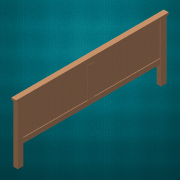
# Autodesk Inventor part: Footer
Saved by Autodesk Inventor 2017 (Build 210142000, 142)
## iProperties
Created: 2017-06-03
Part Number: Footer
Material: Wood (Cherry)
Document SubType Name: Modeling
Designer: Michael
Density: 0.63 g/cm^3
Appearance: Cherry - Natural Low Gloss
Author: Michael
Autodesk Inventor part; units mm, degrees
ref_plane "YZ Plane" through (0, 0, 0) normal (1, 0, 0) x (0, 1, 0)
ref_plane "XZ Plane" through (0, 0, 0) normal (0, 1, 0) x (-1, 0, 0)
ref_plane "XY Plane" through (0, 0, 0) normal (0, 0, 1) x (1, 0, 0)
sketch "Sketch1" plane through (0, 0, 0) normal (0, 1, 0) x (-1, 0, 0)
  line L0 (-23.8125, 804.8625) -> (23.8125, 804.8625)
  line L1 (23.8125, 804.8625) -> (23.8125, 746.125)
  line L2 (23.8125, 746.125) -> (-23.8125, 746.125)
  line L3 (-23.8125, 746.125) -> (-23.8125, 804.8625)
  line L4 (-23.8125, 804.8625) -> (23.8125, 746.125) construction
  line L5 (23.8125, 804.8625) -> (-23.8125, 746.125) construction
  line L6 (-23.8125, -746.125) -> (23.8125, -746.125)
  line L7 (23.8125, -746.125) -> (23.8125, -804.8625)
  line L8 (23.8125, -804.8625) -> (-23.8125, -804.8625)
  line L9 (-23.8125, -804.8625) -> (-23.8125, -746.125)
  line L10 (-23.8125, -746.125) -> (23.8125, -804.8625) construction
  line L11 (23.8125, -746.125) -> (-23.8125, -804.8625) construction
  line L12 (0, 746.125) -> (0, 0) construction
  line L13 (0, 0) -> (0, -746.125) construction
  point P0 (0, 775.4938)
  point P1 (0, -775.4938)
  point P2 (0, 775.4938)
  point P3 (0, -775.4938)
  dimension "d0" = 47.625
  dimension "d1" = 58.7375
  dimension "d2" = 1609.725
  constraints: 28 end point, 8 midpoint, 4 parallel, 3 equal length, 2 horizontal, 2 perpendicular, 2 vertical alignment, 1 point on line, 1 vertical
  measures "d0" distance of L0.start L0.end
  measures "d1" distance of L0.end L1.end
  measures "d2" distance between parallel lines of L8 L0
extrude "Extrusion1" add sketch "Sketch1" along normal blind 635
sketch "Sketch2" plane through (0, 0, 0) normal (0, 0, 1) x (1, 0, 0)
  line L0 (-26.9875, 657.225) -> (26.9875, 657.225)
  line L1 (26.9875, 657.225) -> (26.9875, 635)
  line L2 (26.9875, 635) -> (-26.9875, 635)
  line L3 (-26.9875, 635) -> (-26.9875, 657.225)
  line L4 (-26.9875, 657.225) -> (26.9875, 635) construction
  line L5 (26.9875, 657.225) -> (-26.9875, 635) construction
  line L6 (23.8125, 0) -> (-23.8125, 0) projected
  point P0 (0, 0)
  point P1 (0, 646.1125)
  point P2 (-23.8125, 635)
  point P3 (0, 646.1125)
  point P4 (0, 0)
  dimension "d5" = 53.975
  dimension "d6" = 22.225
  constraints: 12 end point, 4 midpoint, 2 parallel, 1 horizontal, 1 perpendicular, 1 point on line, 1 vertical alignment
  measures "d5" distance of L0.start L0.end
  measures "d6" distance of L0.end L1.end
extrude "Extrusion2" add sketch "Sketch2" along normal mid plane 1651
sketch "Sketch3" plane through (0, 0, 0) normal (0, 0, 1) x (1, 0, 0)
  line L0 (23.8125, 635) -> (-23.8125, 635) projected
  line L1 (11.1125, 581.025) -> (-11.1125, 581.025)
  line L2 (-11.1125, 581.025) -> (-11.1125, 635)
  line L3 (-11.1125, 635) -> (11.1125, 635)
  line L4 (11.1125, 635) -> (11.1125, 581.025)
  line L5 (11.1125, 581.025) -> (-11.1125, 635) construction
  line L6 (-11.1125, 581.025) -> (11.1125, 635) construction
  line L7 (11.1125, 200.025) -> (-11.1125, 200.025)
  line L8 (-11.1125, 200.025) -> (-11.1125, 254)
  line L9 (-11.1125, 254) -> (11.1125, 254)
  line L10 (11.1125, 254) -> (11.1125, 200.025)
  line L11 (11.1125, 200.025) -> (-11.1125, 254) construction
  line L12 (-11.1125, 200.025) -> (11.1125, 254) construction
  point P0 (0, 0)
  point P1 (0, 608.0125)
  point P2 (0, 608.0125)
  point P3 (0, 635)
  point P4 (0, 227.0125)
  point P5 (0, 227.0125)
  dimension "d9" = 53.975
  dimension "d10" = 22.225
  dimension "d11" = 200.025
  constraints: 24 end point, 7 midpoint, 4 parallel, 2 equal length, 2 horizontal, 2 perpendicular, 2 vertical alignment, 1 point on line
  measures "d9" distance of L1.end L2.end
  measures "d10" distance between parallel lines of L2 L4
  measures "d11" distance from line of point (0, 0) L7
extrude "Extrusion3" add sketch "Sketch3" against normal up to surface (1492.25 mm away) from surface at 746.125
sketch "Sketch4" plane through (-11.1125, 254, 746.125) normal (0, 1, 0) x (1, 0, 0)
  line L0 (22.225, 709.6125) -> (0, 709.6125)
  line L1 (0, 709.6125) -> (0, 782.6375)
  line L2 (0, 782.6375) -> (22.225, 782.6375)
  line L3 (22.225, 782.6375) -> (22.225, 709.6125)
  line L4 (22.225, 709.6125) -> (0, 782.6375) construction
  line L5 (0, 709.6125) -> (22.225, 782.6375) construction
  line L6 (5.5562, 0) -> (16.6687, 0)
  line L7 (16.6687, 0) -> (16.6687, 709.6125)
  line L8 (16.6687, 709.6125) -> (5.5562, 709.6125)
  line L9 (5.5562, 709.6125) -> (5.5562, 0)
  line L10 (5.5562, 0) -> (16.6687, 709.6125) construction
  line L11 (16.6687, 0) -> (5.5562, 709.6125) construction
  line L12 (-12.7, 0) -> (34.925, 0) projected
  line L13 (0, 0) -> (0, 1492.25) projected
  line L14 (5.5563, 1492.25) -> (16.6688, 1492.25)
  line L15 (16.6688, 1492.25) -> (16.6688, 782.6375)
  line L16 (16.6688, 782.6375) -> (5.5563, 782.6375)
  line L17 (5.5563, 782.6375) -> (5.5563, 1492.25)
  line L18 (5.5563, 1492.25) -> (16.6688, 782.6375) construction
  line L19 (16.6688, 1492.25) -> (5.5563, 782.6375) construction
  point P0 (11.1125, 746.125)
  point P1 (11.1125, 354.8063)
  point P2 (0, 746.125)
  point P3 (11.1125, 746.125)
  point P4 (11.1125, 1137.4438)
  point P5 (11.1125, 354.8063)
  point P6 (11.1125, 746.125)
  point P7 (11.1125, 1137.4438)
  dimension "d14" = 11.1125
  dimension "d15" = 22.225
  dimension "d16" = 73.025
  constraints: 36 end point, 11 midpoint, 6 parallel, 3 horizontal, 3 perpendicular, 3 point on line, 2 equal length, 2 vertical alignment, 1 horizontal alignment
  measures "d14" distance between parallel lines of L17 L15
  measures "d15" distance of L1.end L2.end
  measures "d16" distance of L0.end L1.end
extrude "Extrusion4" add sketch "Sketch4" along normal up to next separate body contours L0 L1 L2 L3 | L7 L6 L9 L0 | L2 L17 L14 L15
chamfer "Chamfer1" distance 1.5875 angle 45 8 edges at (11.1125, 581.025, 0) (11.1125, 254, 0) (-11.1125, 581.025, 0) (-11.1125, 254, 0) (11.1125, 417.5125, 36.5125) (11.1125, 417.5125, -36.5125) (-11.1125, 417.5125, -36.5125) (-11.1125, 417.5125, 36.5125)
body "Solid1"
body "Solid2"
